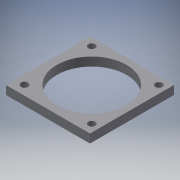
# Autodesk Inventor part: F608Brace
Saved by Autodesk Inventor 2018 (Build 220112000, 112)
## iProperties
Created: 2018-05-15
Part Number: F608Brace
Material: Generic
Document SubType Name: Modeling
Designer: Dan
Density: 1 g/cm^3
Appearance: Default
Author: Dan
Autodesk Inventor part; units mm, degrees
ref_plane "YZ Plane" through (0, 0, 0) normal (1, 0, 0) x (0, 1, 0)
ref_plane "XZ Plane" through (0, 0, 0) normal (0, 1, 0) x (-1, 0, 0)
ref_plane "XY Plane" through (0, 0, 0) normal (0, 0, 1) x (1, 0, 0)
sketch "Sketch1" plane through (0, 0, 0) normal (0, 0, 1) x (1, 0, 0)
  arc A0 (13.944, 13.3501) -> (15.5243, 13.351) centre (14.7334, 14.7418) ccw projected
  line L0 (13.944, 13.3501) -> (13.9333, 13.3543) projected
  line L1 (13.9333, 13.3543) -> (13.9235, 13.3619) projected
  arc A1 (13.1932, 14.3082) -> (13.9235, 13.3619) centre (14.7334, 14.7418) ccw projected
  line L2 (13.1932, 14.3082) -> (13.1833, 14.3294) projected
  line L3 (13.1833, 14.3294) -> (13.1794, 14.3606) projected
  arc A2 (13.1334, 14.7286) -> (13.1794, 14.3606) centre (14.7334, 14.7418) ccw projected
  line L4 (13.1334, 14.7286) -> (13.1333, 14.7294) projected
  line L5 (13.1333, 14.7294) -> (13.1334, 14.7302) projected
  arc A3 (13.1798, 15.1245) -> (13.1334, 14.7302) centre (14.7334, 14.7418) ccw projected
  line L6 (13.1798, 15.1245) -> (13.1833, 15.1544) projected
  line L7 (13.1833, 15.1544) -> (13.1934, 15.176) projected
  arc A4 (15.5428, 13.3616) -> (13.1934, 15.176) centre (14.7334, 14.7418) ccw projected
  line L8 (15.5428, 13.3616) -> (15.5333, 13.3543) projected
  line L9 (15.5333, 13.3543) -> (15.5243, 13.351) projected
  arc A5 (13.9439, -17.6499) -> (15.5243, -17.649) centre (14.7334, -16.2582) ccw projected
  line L10 (13.9439, -17.6499) -> (13.9333, -17.6456) projected
  line L11 (13.9333, -17.6456) -> (13.9235, -17.6381) projected
  arc A6 (13.1932, -16.6917) -> (13.9235, -17.6381) centre (14.7334, -16.2582) ccw projected
  line L12 (13.1932, -16.6917) -> (13.1833, -16.6706) projected
  line L13 (13.1833, -16.6706) -> (13.1795, -16.6395) projected
  arc A7 (13.1334, -16.2713) -> (13.1795, -16.6395) centre (14.7334, -16.2582) ccw projected
  line L14 (13.1334, -16.2713) -> (13.1333, -16.2706) projected
  line L15 (13.1333, -16.2706) -> (13.1334, -16.2699) projected
  arc A8 (13.1798, -15.8754) -> (13.1334, -16.2699) centre (14.7334, -16.2582) ccw projected
  line L16 (13.1798, -15.8754) -> (13.1833, -15.8456) projected
  line L17 (13.1833, -15.8456) -> (13.1934, -15.824) projected
  arc A9 (15.5428, -17.6384) -> (13.1934, -15.824) centre (14.7334, -16.2582) ccw projected
  line L18 (15.5428, -17.6384) -> (15.5333, -17.6457) projected
  line L19 (15.5333, -17.6457) -> (15.5243, -17.649) projected
  arc A10 (-17.0561, 13.3501) -> (-15.4757, 13.3509) centre (-16.2666, 14.7418) ccw projected
  line L20 (-17.0561, 13.3501) -> (-17.0667, 13.3544) projected
  line L21 (-17.0667, 13.3544) -> (-17.0764, 13.3619) projected
  arc A11 (-17.8068, 14.3083) -> (-17.0764, 13.3619) centre (-16.2666, 14.7418) ccw projected
  line L22 (-17.8068, 14.3083) -> (-17.8166, 14.3294) projected
  line L23 (-17.8166, 14.3294) -> (-17.8205, 14.3604) projected
  arc A12 (-17.8666, 14.7288) -> (-17.8205, 14.3604) centre (-16.2666, 14.7418) ccw projected
  line L24 (-17.8666, 14.7288) -> (-17.8667, 14.7294) projected
  line L25 (-17.8667, 14.7294) -> (-17.8666, 14.73) projected
  arc A13 (-17.8201, 15.1247) -> (-17.8666, 14.73) centre (-16.2666, 14.7418) ccw projected
  line L26 (-17.8201, 15.1247) -> (-17.8166, 15.1544) projected
  line L27 (-17.8166, 15.1544) -> (-17.8066, 15.1759) projected
  arc A14 (-15.4571, 13.3617) -> (-17.8066, 15.1759) centre (-16.2666, 14.7418) ccw projected
  line L28 (-15.4571, 13.3617) -> (-15.4667, 13.3543) projected
  line L29 (-15.4667, 13.3543) -> (-15.4757, 13.3509) projected
  circle A15 centre (-13.0857, 32.4807) radius 6.1 projected
  circle A16 centre (48.0582, -36.5955) radius 2.65 projected
  circle A17 centre (-36.5916, 13.2044) radius 2.65 projected
  circle A18 centre (-36.5916, 48.0783) radius 2.65 projected
  circle A19 centre (13.2084, -36.5956) radius 2.65 projected
  circle A20 centre (32.4836, -13.1705) radius 6.1 projected
  circle A21 centre (-0.7667, -0.7706) radius 16.1 projected
  arc A22 (-15.4508, -14.9187) -> (-17.0909, -17.6183) centre (-16.4898, -16.1355) ccw projected
  line L30 (-15.4508, -14.9187) -> (-15.1347, -15.1444) projected
  line L31 (-15.1347, -15.1444) -> (-14.8848, -15.4694) projected
  line L32 (-14.8848, -15.4694) -> (-14.7348, -15.8444) projected
  line L33 (-14.7348, -15.8444) -> (-14.6849, -16.2691) projected
  line L34 (-14.6849, -16.2691) -> (-14.735, -16.6695) projected
  line L35 (-14.735, -16.6695) -> (-14.885, -17.0445) projected
  line L36 (-14.885, -17.0445) -> (-15.135, -17.3694) projected
  line L37 (-15.135, -17.3694) -> (-15.485, -17.6445) projected
  line L38 (-15.485, -17.6445) -> (-15.86, -17.7944) projected
  line L39 (-15.86, -17.7944) -> (-16.26, -17.8444) projected
  line L40 (-16.26, -17.8444) -> (-16.685, -17.7944) projected
  line L41 (-16.685, -17.7944) -> (-17.06, -17.6444) projected
  line L42 (-17.06, -17.6444) -> (-17.0909, -17.6183) projected
  line L43 (-46.8031, 83.2548) -> (-48.8031, 83.2544) projected
  line L44 (-48.8031, 83.2544) -> (-48.7802, -21.5956) projected
  line L45 (-48.7802, -21.5956) -> (-21.5802, -21.5896) projected
  line L46 (-21.5802, -21.5896) -> (-21.5742, -48.7896) projected
  line L47 (-21.5742, -48.7896) -> (83.2758, -48.7667) projected
  line L48 (83.2758, -48.7667) -> (83.2753, -46.7667) projected
  line L49 (83.2753, -46.7667) -> (-46.8031, 83.2548) projected
  line L50 (18.2361, 18.2441) -> (-20.5639, 18.2441)
  line L51 (-20.5639, 18.2441) -> (-20.5639, -20.5729)
  line L52 (-20.5639, -20.5729) -> (18.2361, -20.5729)
  line L53 (18.2361, -20.5729) -> (18.2361, 18.2441)
  circle A23 centre (-0.7667, -0.7706) radius 11.5
  point P0 (0, 0)
  dimension "d0" = 38.8
  dimension "d3" = 23
  constraints: 8 end point, 2 parallel, 1 centre point, 1 coincident, 1 horizontal, 1 midpoint, 1 perpendicular
  measures "d0" distance of L52.end L51.end
  measures "d3" diameter of A23
extrude "Extrusion1" add sketch "Sketch1" along normal blind 4 contours A21 | L53 L52 L51 L50
body "Solid1"
